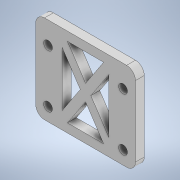
# Autodesk Inventor part: face-2
Saved by Autodesk Inventor 2021 (Build 250183000, 183)
## iProperties
Created: 2024-07-20
Part Number: face-2
Material: Generic
Document SubType Name: Modeling
Designer: Toby
Density: 1 g/cm^3
Appearance: Default
Author: Toby
Autodesk Inventor part; units mm, degrees
ref_plane "YZ Plane" through (0, 0, 0) normal (1, 0, 0) x (0, 1, 0)
ref_plane "XZ Plane" through (0, 0, 0) normal (0, 1, 0) x (-1, 0, 0)
ref_plane "XY Plane" through (0, 0, 0) normal (0, 0, 1) x (1, 0, 0)
sketch "Sketch1" plane through (0, 0, 0) normal (0, 0, 1) x (1, 0, 0)
  line L0 (-20.0276, 11.0224) -> (2.5724, 11.0224)
  line L1 (2.5724, 11.0224) -> (2.5724, -8.9776)
  line L2 (2.5724, -8.9776) -> (-20.0276, -8.9776)
  line L3 (-20.0276, -8.9776) -> (-20.0276, 11.0224)
  line L4 (-14.0276, 9.0224) -> (-3.4276, 9.0224)
  line L5 (-3.4276, 9.0224) -> (-3.4276, -6.9776)
  line L6 (-3.4276, -6.9776) -> (-14.0276, -6.9776)
  line L7 (-14.0276, -6.9776) -> (-14.0276, 9.0224)
  point P0 (0, 0)
  point P1 (-20.0276, -6.9776)
  point P2 (-20.0276, 9.0224)
  point P3 (-18.0276, -6.9776)
  point P4 (-18.0276, 9.0224)
  dimension "d0" = 20
  dimension "d1" = 22.6
  dimension "d2" = 2
  dimension "d3" = 6
  dimension "d4" = 6
  dimension "d5" = 2
  constraints: 16 end point, 4 parallel, 2 horizontal, 2 perpendicular
  measures "d0" distance of L2.end L0.start
  measures "d1" distance of L0.start L0.end
  measures "d2" distance between parallel lines of L4 L0
  measures "d3" distance between parallel lines of L3 L7
  measures "d4" distance between parallel lines of L1 L5
  measures "d5" distance between parallel lines of L2 L6
extrude "Extrusion1" add sketch "Sketch1" along normal blind 2
sketch "Sketch2" plane through (0, 0, 2) normal (0, 0, 1) x (1, 0, 0)
  line L0 (-20.0276, 11.0224) -> (-20.0276, -8.9776) projected
  line L1 (-20.0276, -8.9776) -> (2.5724, -8.9776) projected
  line L2 (2.5724, -8.9776) -> (2.5724, 11.0224) projected
  point P0 (0, 0)
  point P1 (-17.2276, 6.0224)
  point P2 (-17.2276, -5.9776)
  point P3 (-0.2276, 6.0224)
  point P4 (-0.2276, -5.9776)
  dimension "d8" = 2.8
  dimension "d9" = 3
  dimension "d10" = 3
  dimension "d11" = 2.8
  dimension "d12" = 2.8
  dimension "d13" = 2.8
  dimension "d14" = 12
  dimension "d15" = 12
  measures "d8" distance from line of L0 point (-17.228, -5.978)
  measures "d9" distance from line of L1 point (-17.228, -5.978)
  measures "d10" distance from line of L1 point (-0.228, -5.978)
  measures "d11" distance from line of L2 point (-0.228, -5.978)
  measures "d12" distance from line of L0 point (-17.228, 6.022)
  measures "d13" distance from line of L2 point (-0.228, 6.022)
  measures "d14" distance of point (-17.228, -5.978) point (-17.228, 6.022)
  measures "d15" distance of point (-0.228, -5.978) point (-0.228, 6.022)
hole "Hole1" at (-17.2276, 6.0224, 2) at (-17.2276, -5.9776, 2) at (-0.2276, 6.0224, 2) at (-0.2276, -5.9776, 2) direction (0, 0, -1) diameter 2 depth 10 tip angle 118
sketch "Sketch3" plane through (0, 0, 2) normal (0, 0, 1) x (1, 0, 0)
  line L0 (-14.0276, -6.9776) -> (-14.0276, 9.0224) projected
  line L1 (-3.4276, 9.0224) -> (-3.4276, -6.9776) projected
  line L2 (-14.0276, 9.0224) -> (-3.4276, -6.9776) construction
  line L3 (-14.8612, 8.4701) -> (-4.2612, -7.5299)
  line L4 (-2.5939, -6.4253) -> (-13.1939, 9.5747)
  arc A0 (-13.1939, 9.5747) -> (-14.8612, 8.4701) centre (-14.0276, 9.0224) ccw
  arc A1 (-4.2612, -7.5299) -> (-2.5939, -6.4253) centre (-3.4276, -6.9776) ccw
  line L5 (-3.4276, 9.0224) -> (-14.0276, -6.9776) construction
  line L6 (-4.2612, 9.5747) -> (-14.8612, -6.4253)
  line L7 (-13.1939, -7.5299) -> (-2.5939, 8.4701)
  arc A2 (-2.5939, 8.4701) -> (-4.2612, 9.5747) centre (-3.4276, 9.0224) ccw
  arc A3 (-14.8612, -6.4253) -> (-13.1939, -7.5299) centre (-14.0276, -6.9776) ccw
  point P0 (0, 0)
  point P1 (-8.7276, 1.0224)
  point P2 (-8.7276, 1.0224)
  point P3 (-9.9271, 1.0224)
  point P4 (-8.7276, -0.7882)
  point P5 (-7.528, 1.0224)
  point P6 (-8.7276, 2.833)
  dimension "d23" = 2
  dimension "d24" = 2
  constraints: 16 end point, 8 point on circle, 8 tangent, 4 centre point, 2 midpoint, 2 parallel
  measures "d23" diameter of A1
  measures "d24" diameter of A3
extrude "Extrusion2" add sketch "Sketch3" against normal blind 2 contours L6 L3 L7 A3 | L3 A0 L4 L6 | L6 L4 L7 L3 | L7 L4 A1 L3 | L6 A2 L7 L4
fillet "Fillet1" radius 2 4 edges at (-20.0276, 11.0224, 1) (2.5724, 11.0224, 1) (2.5724, -8.9776, 1) (-20.0276, -8.9776, 1)
body "Solid1"
